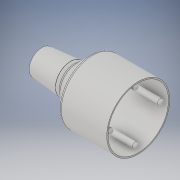
# Autodesk Inventor part: CheckValve 1.0
Saved by Autodesk Inventor 2019 (Build 230136000, 136)
## iProperties
Created: 2019-04-04
Part Number: CheckValve 1.0
Material: Generic
Document SubType Name: Modeling
Designer: Kepler
Density: 1 g/cm^3
Appearance: Default
Author: Kepler
Autodesk Inventor part; units mm, degrees
ref_plane "YZ Plane" through (0, 0, 0) normal (1, 0, 0) x (0, 1, 0)
ref_plane "XZ Plane" through (0, 0, 0) normal (0, 1, 0) x (-1, 0, 0)
sketch "Sketch1" plane through (0, 0, 0) normal (0, 0, 1) x (1, 0, 0)
  line L0 (0, 0) -> (20, 0)
  line L1 (-0.001, 9) -> (21.999, 10.9248)
  line L2 (-0.001, 9) -> (0, 10)
  line L3 (0, 10) -> (22, 11.9248)
  line L4 (26.3004, 11) -> (22.8601, 11)
  line L5 (25.8861, 12) -> (22.8601, 12)
  line L6 (22, 11.9248) -> (22.8601, 12)
  line L7 (21.999, 10.9248) -> (22.8601, 11)
  line L8 (27.3004, 12.5858) -> (39.1288, 24.4142)
  line L9 (40.543, 25) -> (76.543, 25)
  line L10 (27.7146, 11.5858) -> (39.543, 23.4142)
  line L11 (40.9572, 24) -> (76.543, 24)
  line L12 (76.543, 24) -> (76.543, 25)
  arc A0 (40.543, 25) -> (39.1288, 24.4142) centre (40.543, 23) ccw
  arc A1 (40.9572, 24) -> (39.543, 23.4142) centre (40.9572, 22) ccw
  arc A2 (25.8861, 12) -> (27.3004, 12.5858) centre (25.8861, 14) ccw
  arc A3 (26.3004, 11) -> (27.7146, 11.5858) centre (26.3004, 13) ccw
  point P0 (27.1288, 11)
  point P1 (26.7146, 12)
  dimension "d0" = 20
  dimension "d1" = 5
  dimension "d2" = 9
  dimension "d3" = 22
  dimension "d5" = 22
  dimension "d6" = 1
  dimension "d9" = 50
  dimension "d10" = 135
  dimension "d11" = 1
  dimension "d12" = 2
  dimension "d37" = 36
  constraints: 26 end point, 8 point on circle, 8 tangent, 4 centre point, 4 point on line, 3 equal radius, 3 horizontal, 2 parallel, 1 perpendicular
  measures "d0" distance of L0.start L0.end
  measures "d1" angle of L1 L0
  measures "d2" distance of L0.start L1.start
  measures "d3" horizontal distance of L1.start L1.end
  measures "d5" diameter of L4 L0
  measures "d6" distance between parallel lines of L4 L5
  measures "d9" diameter of L9 L0
  measures "d10" angle of L9 L8
  measures "d11" distance between parallel lines of L10 L8
  measures "d12" radius of A0
  measures "d37" distance of L9.start L9.end
revolve "Revolution1" add sketch "Sketch1" angle 360 about axis through (0, 0, 0) along (1, 0, 0)
fillet "Fillet1" radius 2 2 edges at (21.999, -10.9248, 0) (22.8601, -11, 0)
fillet_without_effect "Fillet2"
ref_plane "Work Plane1" through (40.9572, 0, 0) normal (1, 0, 0) x (0, 1, 0)
sketch "Sketch2" plane through (40.9572, 0, 0) normal (1, 0, 0) x (0, 1, 0)
  line L0 (2, 2) -> (2, 24.3322)
  circle A0 centre (0, 0) radius 24.4142 projected
  line L1 (-2, -2) -> (-2, -24.3322)
  line L2 (2, -2) -> (2, -24.3322)
  line L3 (-24.3322, -2) -> (-2, -2)
  line L4 (2, -2) -> (24.3322, -2)
  line L5 (2, 2) -> (24.3322, 2)
  arc A1 (2, 24.3322) -> (-2, 24.3322) centre (0, 0) ccw
  arc A2 (-24.3322, 2) -> (-24.3322, -2) centre (0, 0) ccw
  arc A3 (-2, -24.3322) -> (2, -24.3322) centre (0, 0) ccw
  arc A4 (24.3322, -2) -> (24.3322, 2) centre (0, 0) ccw
  line L6 (-24.3322, 2) -> (-2, 2)
  line L7 (-2, 2) -> (-2, 24.3322)
  arc A5 (-2, 24.3322) -> (-24.3322, 2) centre (0, 0) ccw
  dimension "d14" = 4
  dimension "d15" = 0
  dimension "d16" = 4
  dimension "d17" = 2
  dimension "d18" = 2
  dimension "d19" = 22.3322
  constraints: 16 end point, 10 point on circle, 5 centre point, 5 coincident, 3 vertical, 2 perpendicular, 2 point on line, 1 horizontal, 10 other
  measures "d14" distance between parallel lines of L4 L5
  measures "d15" distance between parallel lines of L2 L0
  measures "d16" distance between parallel lines of L1 L0
  measures "d17" distance from line of point (0, 0) L5
  measures "d18" distance from line of point (0, 0) L0
  measures "d19" distance from line of A1.start L5
extrude "Extrusion1" add sketch "Sketch2" along normal blind 4 contours L5 A0 L4 L2 L1 L3 L6 L7 L0
sketch "Sketch3" plane through (40.9572, 0, 0) normal (1, 0, 0) x (0, 1, 0)
  circle A0 centre (0, 0) radius 1
  dimension "d24" = 2
  constraints: 1 centre point, 1 coincident
  measures "d24" diameter of A0
extrude "Extrusion2" add sketch "Sketch3" along normal blind 8
sketch "Sketch4" plane through (40.9572, 0, 0) normal (-1, 0, 0) x (0, 0, 1)
  circle A0 centre (20, 0) radius 2
  line L0 (23.9165, -2) -> (2, -2) projected
  circle A1 centre (0, -20) radius 2
  circle A2 centre (-20, 0) radius 2
  circle A3 centre (0, 20) radius 2
  point P0 (0, 0)
  dimension "d28" = 4
  dimension "d29" = 4
  dimension "d30" = 4
  dimension "d31" = 20
  dimension "d32" = 20
  dimension "d33" = 20
  dimension "d34" = 20
  constraints: 4 centre point, 1 tangent
  measures "d28" diameter of A1
  measures "d29" diameter of A2
  measures "d30" diameter of A3
  measures "d31" distance of point (0, 0) A3.centre
  measures "d32" distance of point (0, 0) A0.centre
  measures "d33" distance of point (0, 0) A1.centre
  measures "d34" distance of point (0, 0) A2.centre
extrude "Extrusion3" add sketch "Sketch4" against normal blind 35
fillet "Fillet5" radius 1 1 edges at (44.9572, -1, 0)
fillet "Fillet7" radius 2 4 edges at (75.9572, 20, -2) (75.9572, 0, 18) (75.9572, -20, -2) (75.9572, 0, -22)
body "Solid1"
